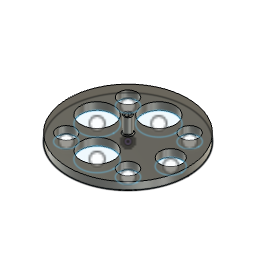
baby-bjorn-wheel (Autodesk Fusion 360 design; units mm, degrees)
Autodesk Fusion 360 part; units mm, degrees
sketch "Sketch1" plane through (0, 0, 0) normal (0, 0, 1) x (1, 0, 0)
  circle A0 centre (0, 0) radius 60
  circle A1 centre (43, 0) radius 11.05
  circle A2 centre (0, 31) radius 16.5
  circle A3 centre (-31, 0) radius 16.5
  circle A4 centre (0, -31) radius 16.5
  circle A5 centre (-31, 31) radius 9
  circle A6 centre (-31, -31) radius 9
  circle A7 centre (31, -31) radius 9
  circle A8 centre (31, 31) radius 9
  dimension "d1" = 120
  dimension "d3" = 22.1
  dimension "d4" = 43
  dimension "d8" = 33
  dimension "d9" = 31
  dimension "d12" = 31
  dimension "d13" = 31
  dimension "d17" = 18
  constraint coincident A0.centre origin
  measures "d1" diameter of A0
  measures "d3" diameter of A1
  measures "d4" distance of A0.centre A1.centre
  measures "d8" diameter of A2
  measures "d9" distance of A0.centre A2.centre
  measures "d12" horizontal distance of A2.centre A5.centre
  measures "d13" vertical distance of A3.centre A5.centre
  measures "d17" diameter of A5
extrude "Extrude2" add sketch "Sketch1" along normal blind 7.5
sketch "Sketch2" plane through (0, 0, 7.5) normal (0, 0, 1) x (-1, 0, 0)
  circle A0 centre (31, -31) radius 9
  circle A1 centre (0, 31) radius 16.5
  circle A2 centre (-31, -31) radius 9
  circle A3 centre (31, 0) radius 16.5
  circle A4 centre (0, -31) radius 16.5
  circle A5 centre (-31, 31) radius 9
  circle A6 centre (-43, 0) radius 11.05
  circle A7 centre (31, 31) radius 9
  circle A8 centre (0, 0) radius 60
  circle A9 centre (0, 0) radius 3.95
  dimension "d20" = 7.9
  constraint concentric A8 A9
  measures "d20" diameter of A9
extrude "Extrude3" add sketch "Sketch2" along normal blind 16 contours A9
sketch "Sketch3" plane through (0, 0, 23.5) normal (0, 0, 1) x (-1, 0, 0)
  circle A0 centre (0, 0) radius 3.95
  circle A1 centre (0, 0) radius 2.85
  line L0 (-1.925, 5) -> (1.925, 5)
  line L1 (1.925, 5) -> (1.925, -5)
  line L2 (1.925, -5) -> (-1.925, -5)
  line L3 (-1.925, -5) -> (-1.925, 5)
  line L4 (-1.925, 5) -> (1.925, -5) construction
  line L5 (1.925, 5) -> (-1.925, -5) construction
  dimension "d23" = 5.7
  dimension "d24" = 3.85
  dimension "d25" = 10
  constraint coincident A0.centre A1.centre
  constraint horizontal L0
  constraint perpendicular L0 L1
  constraint parallel L0 L2
  constraint parallel L1 L3
  constraint coincident L4 A0.centre
  constraint coincident L5 A0.centre
  measures "d23" diameter of A1
  measures "d24" distance of L1.end L2.end
  measures "d25" distance of L0.end L1.end
extrude "Extrude4" cut sketch "Sketch3" against normal blind 8 contours A1 L1 L3
fillet "Fillet1" radius 1 1 edges at (3.6827, -1.4284, 7.5)
equation "tol1 = 0.1 mm"
equation "d3 = 22 mm + tol1"
equation "d12 = ho1"
equation "d13 = ho1"
equation "ho1 = 31 mm"
equation "d20 = 8 mm - tol1"
equation "d21 = 7 mm + 7 mm + 2 mm"
equation "d23 = 5.6 mm + tol1"
equation "d24 = 3.75 mm + tol1"
